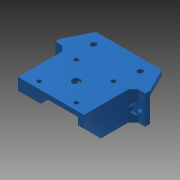
# Autodesk Inventor part: ZMotorMount
Saved by Autodesk Inventor 2016 (Build 200138000, 138)
## iProperties
Category: Print
Created: 2015-01-11
Part Number: ZMotorMount
Material: ABS Plastic
Document SubType Name: Modeling
Designer: Jack
Density: 1.06 g/cm^3
Appearance: Cyan
Mass: 25.3831 g
Surface Area: 133.839 cm^2
Volume: 23.9464 cm^3
Vendor: Jack
Author: Jack
Title: Z Motor Mount
Autodesk Inventor part; units mm, degrees
ref_plane "YZ Plane" through (0, 0, 0) normal (1, 0, 0) x (0, 1, 0)
ref_plane "XZ Plane" through (0, 0, 0) normal (0, 1, 0) x (-1, 0, 0)
ref_plane "XY Plane" through (0, 0, 0) normal (0, 0, 1) x (1, 0, 0)
sketch "Sketch1" plane through (0, 0, 0) normal (0, 0, 1) x (1, 0, 0)
  line L0 (0, 0) -> (55, 0)
  line L1 (55, 0) -> (55, 65)
  line L2 (55, 65) -> (0, 65)
  line L3 (0, 65) -> (0, 0)
  dimension "d0" = 55
  dimension "d1" = 65
  constraints: 8 end point, 2 perpendicular, 1 horizontal, 1 vertical
  measures "d0" distance of L0.start L0.end
  measures "d1" distance of L0.end L1.end
extrude "Extrusion1" add sketch "Sketch1" along normal blind 4
sketch "Sketch2" plane through (0, 0, 0) normal (0, 0, -1) x (-1, 0, 0)
  line L0 (0, 0) -> (-55, 0) projected
  line L1 (-55, 65) -> (0, 65) projected
  line L2 (-55, 0) -> (-55, 65) projected
  line L3 (0, 65) -> (0, 0) projected
  line L4 (0, 45) -> (-5, 45)
  line L5 (-5, 45) -> (-5, 0)
  line L6 (-55, 45) -> (-50, 45)
  line L7 (-50, 45) -> (-50, 0)
  dimension "d4" = 5
  dimension "d5" = 20
  constraints: 8 end point, 6 point on line, 3 perpendicular, 1 collinear
  measures "d4" distance of L6.start L6.end
  measures "d5" distance between parallel lines of L1 L4
extrude "Extrusion2" add sketch "Sketch2" along normal blind 20 contours L0 L5 L4 L3 | L0 L2 L6 L7
sketch "Sketch3" plane through (0, 0, 4) normal (-1, 0, 0) x (0, 0, 1)
  line L0 (-4, 65) -> (-4, 45) projected
  line L1 (-4, 45) -> (-24, 45) projected
  line L2 (-4, 45) -> (-4, 41)
  line L3 (-4, 41) -> (-24, 41)
  line L4 (-24, 45) -> (-24, 0) projected
  point P0 (-4, 0)
  dimension "d8" = 4
  constraints: 4 end point, 2 point on line, 1 perpendicular
  measures "d8" distance of L0.end L2.end
extrude "Extrusion3" add sketch "Sketch3" along normal blind 10
sketch "Sketch4" plane through (55, 0, 4) normal (1, 0, 0) x (0, 0, -1)
  line L0 (24, 45) -> (24, 0) projected
  line L1 (4, 45) -> (24, 45) projected
  line L2 (4, 41) -> (24, 41) projected
  line L3 (4, 41) -> (4, 45) projected
  point P0 (4, 0)
extrude "Extrusion4" add sketch "Sketch4" along normal blind 10
sketch "Sketch5" plane through (0, 0, 0) normal (0, 0, -1) x (-1, 0, 0)
  line L0 (-5, 0) -> (-50, 0) projected
  line L1 (-5, 0) -> (-5, 45) projected
  circle A0 centre (-12, 5.65) radius 1.75
  circle A1 centre (-12, 36.65) radius 1.75
  circle A2 centre (-43, 5.65) radius 1.75
  circle A3 centre (-43, 36.65) radius 1.75
  point P0 (0, 0)
  dimension "d13" = 3.5
  dimension "d14" = 31
  dimension "d15" = 31
  dimension "d16" = 7
  dimension "d17" = 5.65
  constraints: 4 centre point, 3 equal radius, 2 horizontal alignment, 2 vertical alignment
  measures "d13" diameter of A0
  measures "d14" distance of A2.centre A0.centre
  measures "d15" distance of A1.centre A0.centre
  measures "d16" distance from line of L1 A0.centre
  measures "d17" distance from line of L0 A0.centre
extrude "Extrusion5" cut sketch "Sketch5" against normal up to next
chamfer "Chamfer1" distance 14 angle 45 2 edges at (2.5, 0, -20) (52.5, 0, -20)
sketch "Sketch6" plane through (0, 0, 4) normal (0, 0, 1) x (1, 0, 0)
  line L0 (55, 0) -> (55, 65) projected
  line L1 (55, 65) -> (0, 65) projected
  line L2 (0, 65) -> (0, 0) projected
  circle A0 centre (8, 55) radius 2.25
  circle A1 centre (47, 55) radius 2.25
  dimension "d23" = 4.5
  dimension "d24" = 10
  dimension "d25" = 8
  dimension "d26" = 8
  constraints: 2 centre point, 1 equal radius, 1 horizontal alignment
  measures "d23" diameter of A0
  measures "d24" distance from line of L1 A0.centre
  measures "d25" distance from line of L0 A1.centre
  measures "d26" distance from line of L2 A0.centre
extrude "Extrusion6" cut sketch "Sketch6" against normal up to next
sketch "Sketch7" plane through (0, 41, -20) normal (0, -1, 0) x (1, 0, 0)
  line L0 (0, 20) -> (-10, 20) projected
  line L1 (-10, 0) -> (-10, 20) projected
  line L2 (55, 0) -> (55, 20) projected
  line L3 (55, 0) -> (65, 0) projected
  line L4 (65, 20) -> (65, 0) projected
  line L5 (55, 20) -> (65, 20) projected
  circle A0 centre (-5, 10) radius 2.25
  circle A1 centre (60, 10) radius 2.25
  dimension "d29" = 4.5
  dimension "d30" = 5
  dimension "d31" = 10
  dimension "d32" = 5
  constraints: 2 centre point, 1 equal radius, 1 horizontal alignment
  measures "d29" diameter of A0
  measures "d30" distance from line of L1 A0.centre
  measures "d31" distance from line of L0 A0.centre
  measures "d32" distance from line of L4 A1.centre
extrude "Extrusion7" cut sketch "Sketch7" against normal up to next contours A0 | A1
sketch "Sketch8" plane through (0, 41, 0) normal (0, 0, 1) x (1, 0, 0)
  line L0 (0, 4) -> (0, 0) projected
  line L1 (0, 4) -> (-10, 4) projected
  line L2 (-10, 0) -> (-10, 4) projected
  line L3 (0, 0) -> (-10, 0) projected
  line L4 (55, 0) -> (55, 4) projected
  line L5 (55, 0) -> (65, 0) projected
  line L6 (65, 4) -> (65, 0) projected
  line L7 (55, 4) -> (65, 4) projected
  point P0 (0, -41)
extrude "Extrusion8" add sketch "Sketch8" along normal up to surface (4 mm away)
sketch "Sketch9" plane through (0, 0, 4) normal (0, 0, 1) x (1, 0, 0)
  line L0 (55, 45) -> (65, 45) projected
  line L1 (55, 45) -> (55, 65) projected
  line L2 (0, 65) -> (0, 45) projected
  line L3 (-10, 45) -> (0, 45) projected
  line L4 (55, 65) -> (65, 45)
  line L5 (0, 65) -> (-10, 45)
  constraints: 4 end point
extrude "Extrusion9" add sketch "Sketch9" against normal blind 4
sketch "Sketch10" plane through (0, 0, 0) normal (0, 0, -1) x (-1, 0, 0)
  circle A0 centre (-43, 5.65) radius 1.75 projected
  circle A1 centre (-27.5, 21.15) radius 12
  point P0 (0, 0)
  dimension "d39" = 24
  dimension "d40" = 15.5
  dimension "d41" = 15.5
  constraints: 1 centre point
  measures "d39" diameter of A1
  measures "d40" horizontal distance of A0.centre A1.centre
  measures "d41" horizontal distance of A0.centre A1.centre
extrude "Extrusion10" cut sketch "Sketch10" against normal blind 2 contours A1
sketch "Sketch11" plane through (27.5, 21.15, 2) normal (0, 0, -1) x (-1, 0, 0)
  circle A0 centre (0, 0) radius 12 projected
  circle A1 centre (0, 0) radius 3.25
  point P0 (27.5, -21.15)
  dimension "d44" = 6.5
  constraints: 1 centre point, 1 coincident
  measures "d44" diameter of A1
extrude "Extrusion11" cut sketch "Sketch11" against normal up to next contours A1
chamfer "Chamfer2" distance 4 angle 45 2 edges at (0, 41, -8) (55, 41, -8)
sketch "Sketch12" plane through (-10, 41, -20) normal (0, -1, 0) x (1, 0, 0)
  arc A0 (6, 12.0156) -> (6, 7.9844) centre (5, 10) ccw projected
  line L0 (69, 12.0156) -> (69, 24) projected
  arc A1 (69, 7.9844) -> (69, 12.0156) centre (70, 10) ccw projected
  line L1 (69, 0) -> (69, 7.9844) projected
  line L2 (69, 0) -> (75, 0) projected
  line L3 (75, 0) -> (75, 24) projected
  line L4 (75, 24) -> (69, 24) projected
  circle A2 centre (5, 10) radius 5
  circle A3 centre (70, 10) radius 5
  point P0 (10, 20)
  dimension "d50" = 10
  dimension "d51" = 10
  constraints: 2 centre point, 2 coincident
  measures "d50" diameter of A2
  measures "d51" diameter of A3
extrude "Extrusion12" cut sketch "Sketch12" along normal blind 7.5 contours A1 L1 A3 L0 | L0 A3 L1 A1 | A2
body "Solid1"
